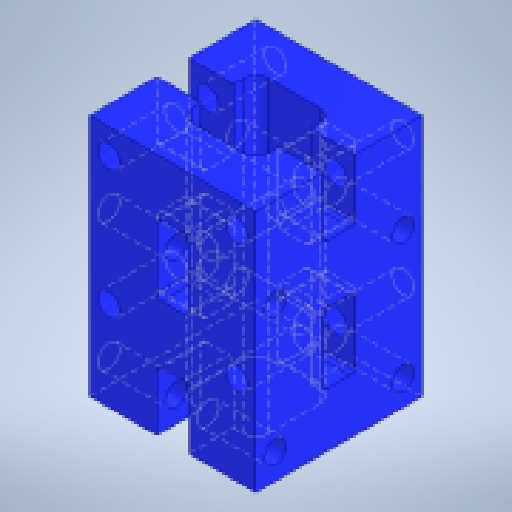
# Autodesk Inventor part: carriage_v1
Saved by Autodesk Inventor 2025 (Build 290162000, 162)
## iProperties
Created: 2025-02-24
Part Number: carriage_v1
Material: ABS プラスチック
Document SubType Name: Modeling
Designer: Zhopa
Density: 1.06 g/cm^3
Appearance: 青 - 壁塗料 - 光沢
Mass: 16.8327 g
Surface Area: 88.1605 cm^2
Volume: 15.8799 cm^3
Author: Zhopa
Autodesk Inventor part; units mm, degrees
ref_plane "YZ Plane" through (0, 0, 0) normal (1, 0, 0) x (0, 1, 0)
ref_plane "XZ Plane" through (0, 0, 0) normal (0, 1, 0) x (-1, 0, 0)
ref_plane "XY Plane" through (0, 0, 0) normal (0, 0, 1) x (1, 0, 0)
sketch "Sketch1" plane through (0, 0, 0) normal (0, 1, 0) x (-1, 0, 0)
  line L0 (5, 5) -> (-5, 5)
  line L1 (-5, 5) -> (-5, -5)
  line L2 (-5, -5) -> (5, -5)
  line L3 (5, -5) -> (5, 5)
  line L4 (5, 5) -> (-5, -5) construction
  line L5 (-5, 5) -> (5, -5) construction
  line L6 (15, 0) -> (15, -2)
  line L7 (15, -2) -> (5, -2)
  line L8 (5, -2) -> (5, 0)
  line L9 (15, 0) -> (15, 2)
  line L10 (15, 2) -> (5, 2)
  line L11 (-13, 13) -> (13, 13)
  line L12 (13, 13) -> (13, -13)
  line L13 (13, -13) -> (-13, -13)
  line L14 (-13, -13) -> (-13, 13)
  line L15 (-13, 13) -> (13, -13) construction
  line L16 (13, 13) -> (-13, -13) construction
  point P0 (0, 0)
  point P1 (10, 0)
  point P2 (13, 0)
  dimension "d0" = 10
  dimension "d1" = 10
  dimension "d2" = 10
  dimension "d3" = 2
  dimension "d4" = 5
  dimension "d5" = 2
  dimension "d6" = 3
  dimension "d7" = 3
  constraints: 34 end point, 5 midpoint, 5 parallel, 2 horizontal, 2 perpendicular, 1 point on line
  measures "d0" distance of L2.end L1.end
  measures "d1" distance of L2.end L0.start
  measures "d2" distance of L6.end L7.end
  measures "d3" distance of L6.start L6.end
  measures "d4" distance from line of L3 point (10, 0)
  measures "d5" distance from line of L7 point (0, 0)
  measures "d6" distance of point (10, 0) point (13, 0)
  measures "d7" distance from line of L12 point (10, 0)
extrude "Extrusion1" add sketch "Sketch1" along normal blind 38 contours L0 L1 L2 L3 L7 L12 L13 L14 L11 L10 | L10 L12 L7 L3
sketch "Sketch2" plane through (0, 0, 0) normal (1, 0, 0) x (0, 1, 0)
  line L0 (0, -13) -> (0, 13) projected
  line L1 (0, 5) -> (38, 5) projected
  line L2 (0, -5) -> (38, -5) projected
  line L3 (0, -13) -> (38, -13) projected
  circle A0 centre (4, 10) radius 1.75
  line L4 (-1.5, 15) -> (9.5, 15)
  line L5 (9.5, 15) -> (9.5, 5)
  line L6 (9.5, 5) -> (-1.5, 5)
  line L7 (-1.5, 5) -> (-1.5, 15)
  line L8 (-1.5, 15) -> (9.5, 5) construction
  line L9 (9.5, 15) -> (-1.5, 5) construction
  line L10 (0, 0) -> (20.9563, 0)
  circle A1 centre (14, 10) radius 1.75
  circle A2 centre (24, 10) radius 1.75
  line L11 (18.5, 15) -> (29.5, 15)
  line L12 (29.5, 15) -> (29.5, 5)
  line L13 (29.5, 5) -> (18.5, 5)
  line L14 (18.5, 5) -> (18.5, 15)
  line L15 (18.5, 15) -> (29.5, 5) construction
  line L16 (29.5, 15) -> (18.5, 5) construction
  circle A3 centre (4, -10) radius 1.75
  line L17 (-1.5, -15) -> (9.5, -15)
  line L18 (9.5, -15) -> (9.5, -5)
  line L19 (9.5, -5) -> (-1.5, -5)
  line L20 (-1.5, -5) -> (-1.5, -15)
  circle A4 centre (24, -10) radius 1.75
  line L21 (18.5, -15) -> (29.5, -15)
  line L22 (29.5, -15) -> (29.5, -5)
  line L23 (29.5, -5) -> (18.5, -5)
  line L24 (18.5, -5) -> (18.5, -15)
  line L25 (39, 2.5) -> (29, 2.5)
  line L26 (29, 2.5) -> (29, -2.5)
  line L27 (29, -2.5) -> (39, -2.5)
  line L28 (39, -2.5) -> (39, 2.5)
  line L29 (39, 2.5) -> (29, -2.5) construction
  line L30 (29, 2.5) -> (39, -2.5) construction
  line L31 (19, 2.5) -> (9, 2.5)
  line L32 (9, 2.5) -> (9, -2.5)
  line L33 (9, -2.5) -> (19, -2.5)
  line L34 (19, -2.5) -> (19, 2.5)
  line L35 (19, 2.5) -> (9, -2.5) construction
  line L36 (9, 2.5) -> (19, -2.5) construction
  line L37 (29, -2.5) -> (28.5, -2.5)
  line L38 (28.5, -2.5) -> (28.5, 2.5)
  line L39 (28.5, 2.5) -> (29, 2.5)
  line L40 (29, 2.5) -> (29, -2.5)
  line L41 (8.5, 2.75) -> (19.5, 2.75)
  line L42 (19.5, 2.75) -> (19.5, -2.75)
  line L43 (19.5, -2.75) -> (8.5, -2.75)
  line L44 (8.5, -2.75) -> (8.5, 2.75)
  line L45 (8.5, 2.75) -> (19.5, -2.75) construction
  line L46 (19.5, 2.75) -> (8.5, -2.75) construction
  line L47 (19, -2.5) -> (19.5, -2.5)
  line L48 (19, 2.5) -> (19.5, 2.5)
  line L49 (9, -2.5) -> (8.5, -2.5)
  line L50 (9, 2.5) -> (8.5, 2.5)
  point P0 (0, 0)
  point P1 (0, 0)
  point P2 (0, 10)
  point P3 (34, 10)
  point P4 (14, 0)
  point P5 (34, 0)
  point P6 (9.5, -13)
  point P7 (9.5, -5)
  point P8 (18.5, -5)
  point P9 (18.5, -13)
  point P10 (29.5, -13)
  point P11 (29.5, -5)
  point P12 (18.5, 5)
  point P13 (9, 0)
  point P14 (19, 0)
  dimension "d10" = 5
  dimension "d11" = 13
  dimension "d12" = 5
  dimension "d13" = 4
  dimension "d14" = 3.5
  dimension "d15" = 0
  dimension "d16" = 11
  dimension "d17" = 10
  dimension "d18" = 10
  dimension "d19" = 3.5
  dimension "d20" = 10
  dimension "d21" = 3.5
  dimension "d22" = 11
  dimension "d23" = 10
  dimension "d24" = 10
  dimension "d25" = 10
  dimension "d26" = 5
  dimension "d27" = 10
  dimension "d43" = 5
  dimension "d44" = 2.5
  dimension "d51" = 0.5
  dimension "d52" = 11
  constraints: 94 end point, 12 parallel, 12 point on line, 11 midpoint, 10 symmetric about line, 7 horizontal, 7 perpendicular, 5 centre point, 5 coincident, 2 other
  measures "d10" distance of L10.start L1.start
  measures "d11" distance of L10.start L0.end
  measures "d12" distance of L1.start point (0, 10)
  measures "d13" distance from line of L0 point (4, 10)
  measures "d14" diameter of A0
  measures "d15" vertical distance of point (0, 10) point (4, 10)
  measures "d16" distance of L5.end L6.end
  measures "d17" distance of L4.end L5.end
  measures "d18" distance of point (4, 10) point (14, 10)
  measures "d19" diameter of A1
  measures "d20" distance of point (14, 10) point (24, 10)
  measures "d21" diameter of A2
  measures "d22" distance of L12.end L13.end
  measures "d23" distance from line of L10 point (14, 10)
  measures "d24" distance of point (34, 10) point (24, 10)
  measures "d25" distance of L27.end L26.end
  measures "d26" distance of L26.end L25.end
  measures "d27" distance of L33.end L32.end
  measures "d43" distance of L33.end L31.start
  measures "d44" distance from line of L10.end L27
  measures "d51" distance of L38.end L39.end
  measures "d52" distance of L42.end L43.end
extrude "Extrusion2" cut sketch "Sketch2" along normal mid plane 5 contours L0 L2 L18 L3 | L14 L11 L12 L1 | L6 L7 L4 L5 L1 | L24 L2 L22 L3
extrude "Extrusion3" cut sketch "Sketch2" along normal mid plane 53 contours A0 | A2 | A3 | A4
extrude "Extrusion4" cut sketch "Sketch2" along normal mid plane 53 contours L32 L31 L34 L10 | L10 L34 L33 L32 | L28 L27 L26 L25
sketch "Sketch3" plane through (-5, 9, 2.5) normal (0, 0, -1) x (-1, 0, 0)
  line L0 (8, 10) -> (8, 0) projected
  line L1 (0, 0) -> (0, 10) projected
  line L2 (8, 10) -> (0, 10) projected
  line L3 (0, 20) -> (0, 29) projected
  line L4 (0, 20) -> (8, 20) projected
  circle A0 centre (5, 25) radius 1.75
  circle A1 centre (5, 5) radius 1.75
  line L5 (-7.5, 0.5) -> (-2.5, 0.5) projected
  line L6 (-5, 0.5) -> (-5, 17.2695)
  circle A2 centre (-15, 25) radius 1.75
  circle A3 centre (-15, 5) radius 1.75
  point P0 (-5, -9)
  dimension "d35" = 5
  dimension "d36" = 5
  dimension "d37" = 5
  dimension "d38" = 5
  dimension "d39" = 3.5
  dimension "d40" = 3.5
  constraints: 4 centre point, 4 coincident, 4 symmetric about line, 2 end point, 1 midpoint, 1 vertical, 2 other
  measures "d35" distance from line of L1 point (5, 5)
  measures "d36" distance from line of L2 point (5, 5)
  measures "d37" distance from line of point (5, 25) L3
  measures "d38" distance from line of L4 point (5, 25)
  measures "d39" diameter of A0
  measures "d40" diameter of A1
extrude "Extrusion5" cut sketch "Sketch3" along normal mid plane 53
sketch "Sketch4" plane through (0, 38, 0) normal (0, 1, 0) x (1, 0, 0)
  line L0 (6, -6) -> (-6, -6)
  line L1 (-6, -6) -> (-6, 6)
  line L2 (-6, 6) -> (6, 6)
  line L3 (6, 6) -> (6, -6)
  line L4 (6, -6) -> (-6, 6) construction
  line L5 (-6, -6) -> (6, 6) construction
  point P0 (0, 0)
  dimension "d45" = 12
  dimension "d46" = 12
  constraints: 12 end point, 2 midpoint, 2 parallel, 1 horizontal, 1 perpendicular
  measures "d45" distance of L1.end L2.end
  measures "d46" distance of L0.end L1.end
extrude "Extrusion6" cut sketch "Sketch4" against normal blind 53
fillet "Fillet1" radius 2 4 edges at (-6, 19, -6) (6, 19, -6) (-6, 19, 6) (6, 19, 6)
extrude "Extrusion7" cut sketch "Sketch2" along normal mid plane 53 contours L44 L50 L32 L10 | L10 L32 L49 L44 | L34 L48 L42 L10 | L10 L42 L47 L34 | L26 L37 L38 L39
fillet "Fillet3" radius 0.74 24 edges at (-9.5, 28.5, -2.5) (9.5, 28.5, -2.5) (-9.5, 28.5, 2.5) (9.5, 28.5, 2.5) (-9.5, 19.5, -2.5) (9.5, 19.5, -2.5) (-9.5, 19.5, 2.5) (9.5, 19.5, 2.5) (-9.5, 8.5, -2.5) (9.5, 8.5, -2.5) (-9.5, 8.5, 2.5) (9.5, 8.5, 2.5) (2.5, 29.5, 9.5) (-2.5, 29.5, 9.5) (-2.5, 18.5, 9.5) (2.5, 18.5, 9.5) (2.5, 9.5, 9.5) (-2.5, 9.5, 9.5) (2.5, 29.5, -9.5) (-2.5, 29.5, -9.5) (-2.5, 18.5, -9.5) (2.5, 18.5, -9.5) (-2.5, 9.5, -9.5) (2.5, 9.5, -9.5)
sketch "Sketch5" plane through (-13, 0, -13) normal (-1, 0, 0) x (0, 0, 1)
  point P0 (13, 0)
equation "\"d7\" = d6"
equation "\"d44\" = 0.5 * d43"
body "Solid1"
